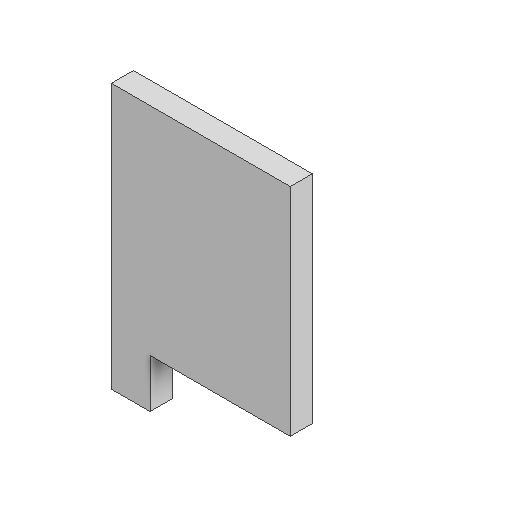
# Autodesk Inventor part: 30_XY_Sample_lightsheetarm_sample_lid
Saved by Autodesk Inventor 2022 (Build 260153000, 153)
## iProperties
Created: 2021-11-10
Part Number: 30_XY_Sample_lightsheetarm_sample_lid
Material: Generic
Document SubType Name: Modeling
Designer: diederichbenedict
Density: 1 g/cm^3
Appearance: Default
Author: diederichbenedict
Autodesk Inventor part; units mm, degrees
ref_plane "YZ Plane" through (0, 0, 0) normal (1, 0, 0) x (0, 1, 0)
ref_plane "XZ Plane" through (0, 0, 0) normal (0, 1, 0) x (-1, 0, 0)
ref_plane "XY Plane" through (0, 0, 0) normal (0, 0, 1) x (1, 0, 0)
sketch "Sketch1" plane through (0, 0, 0) normal (0, 0, 1) x (1, 0, 0)
  line L0 (-3.5, 0) -> (-3.5, -20) projected
  line L1 (-3.5, -20) -> (0, -20) projected
  line L2 (-16.2, -20) -> (-16.2, 4) projected
  line L3 (-16.2, -20) -> (-12.7, -20) projected
  line L4 (-12.7, 0) -> (-12.7, -20) projected
  line L5 (0, 4) -> (-16.2, 4)
  line L6 (-16.2, 4) -> (-16.2, -15.5962)
  line L7 (-16.2, -15.5962) -> (0, -15.5962)
  line L8 (0, -15.5962) -> (0, 4)
  line L9 (0, -20) -> (0, 4) projected
  line L10 (-16.2, 4) -> (0, 4) projected
  line L11 (-12.7, 0) -> (-3.5, 0) projected
  point P0 (0, 0)
  point P1 (-12.7, -15.5962)
  point P2 (-3.5, -15.5962)
  constraints: 8 end point, 2 parallel, 1 horizontal, 1 perpendicular, 1 point on line
extrude "Extrusion1" add sketch "Sketch1" along normal blind 2 contours L11 L4 L7 L2 L5 L8 L0 | L0 L7 L4 L11 | L4 L3 L2 L7
sketch "Sketch2" plane through (0, 0, 2) normal (0, 0, 1) x (1, 0, 0)
  line L0 (0, -15.5962) -> (0, 4) projected
  line L1 (0, 4) -> (-16.2, 4) projected
  line L2 (-16.2, 4) -> (-16.2, -20) projected
  line L3 (-12.7, -15.5962) -> (0, -15.5962) projected
  circle A0 centre (-8.1, -11.6475) radius 1
  line L4 (-12.7, -20) -> (-12.7, -15.5962) projected
  line L5 (-16.2, -20) -> (-12.7, -20) projected
  point P0 (0, 0)
  dimension "d2" = 2
  constraints: 1 centre point
  measures "d2" diameter of A0
extrude "Extrusion2" add sketch "Sketch2" against normal blind 10 contours A0
chamfer "Chamfer1" distance 1 angle 45 1 edges at (-9.1, -11.6475, -8)
pattern_linear "Rectangular Pattern1" [suppressed]
body "Solid1"
